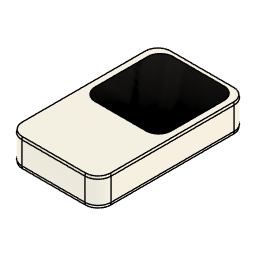
powerbank (Autodesk Fusion 360 design; units mm, degrees)
part number: 2025-04-07-12-48-19-748
Autodesk Fusion 360 part; units mm, degrees
note: some values were not read from the file. Chosen so that the rebuilt part matches the saved one: which bodies a step acts on.
sketch "Szkic1" plane through (0, 0, 0) normal (0, 0, 1) x (1, 0, 0)
  line L0 (-25, 58.75) -> (25, 58.75)
  line L1 (35, 48.75) -> (35, -48.75)
  line L2 (25, -58.75) -> (-25, -58.75)
  line L3 (-35, -48.75) -> (-35, 48.75)
  line L4 (-35, 58.75) -> (35, -58.75) construction
  line L5 (35, 58.75) -> (-35, -58.75) construction
  arc A0 (35, 48.75) -> (25, 58.75) centre (25, 48.75) ccw
  arc A1 (-25, 58.75) -> (-35, 48.75) centre (-25, 48.75) ccw
  arc A2 (-35, -48.75) -> (-25, -58.75) centre (-25, -48.75) ccw
  arc A3 (25, -58.75) -> (35, -48.75) centre (25, -48.75) ccw
  dimension "d1" = 70
  dimension "d2" = 117.5
  dimension "d3" = 10
  constraint horizontal L0
  constraint perpendicular L0 L1
  constraint parallel L0 L2
  constraint parallel L1 L3
  constraint coincident L4 origin
  constraint coincident L5 origin
  constraint coincident L5.start L1
  constraint coincident L5.start L0
  constraint tangent L1 A0
  constraint tangent L0 A0
  constraint coincident L4.start L0
  constraint coincident L4.start L3
  constraint tangent L0 A1
  constraint tangent L3 A1
  constraint equal A0 A1
  constraint coincident L5.end L3
  constraint coincident L5.end L2
  constraint tangent L3 A2
  constraint tangent L2 A2
  constraint equal A0 A2
  constraint coincident L4.end L2
  constraint coincident L4.end L1
  constraint tangent L2 A3
  constraint tangent L1 A3
  constraint equal A0 A3
  measures "d1" distance of L4.end L5.end
  measures "d2" distance of L5.start L4.end
  measures "d3" radius of A0
extrude "Wyciągnięcie proste4" add sketch "Szkic1" along normal blind 2 draft 10 makes body 1
extrude "Wyciągnięcie proste5" add 1 faces at (11.7842, -16.25, 2) along direction (0, 0, 1) blind 18 on bodies 1 bodies 1
extrude "Wyciągnięcie proste6" add 1 faces at (11.7842, -16.25, 20) along direction (0, 0, 1) blind 2 draft -10 on bodies 1 bodies 1
sketch "Szkic3" plane through (0, 0, 22) normal (0, 0, 1) x (-1, 0, 0)
  line L0 (35, -48.75) -> (35, 48.75)
  arc A0 (35, 48.75) -> (25, 58.75) centre (25, 48.75) ccw
  line L1 (25, 58.75) -> (-25, 58.75)
  arc A1 (-25, 58.75) -> (-35, 48.75) centre (-25, 48.75) ccw
  line L2 (-35, 48.75) -> (-35, -48.75)
  arc A2 (-35, -48.75) -> (-25, -58.75) centre (-25, -48.75) ccw
  line L3 (-25, -58.75) -> (25, -58.75)
  arc A3 (25, -58.75) -> (35, -48.75) centre (25, -48.75) ccw
  line L4 (-20.1713, -55.8211) -> (20.1713, -55.8211)
  line L5 (30.1713, -45.8211) -> (30.1713, -4.1789)
  line L6 (20.1713, 5.8211) -> (-20.1713, 5.8211)
  line L7 (-30.1713, -4.1789) -> (-30.1713, -45.8211)
  line L8 (-30.1713, -55.8211) -> (30.1713, 5.8211) construction
  line L9 (30.1713, -55.8211) -> (-30.1713, 5.8211) construction
  arc A4 (20.1713, -55.8211) -> (30.1713, -45.8211) centre (20.1713, -45.8211) ccw
  arc A5 (-30.1713, -45.8211) -> (-20.1713, -55.8211) centre (-20.1713, -45.8211) ccw
  arc A6 (-20.1713, 5.8211) -> (-30.1713, -4.1789) centre (-20.1713, -4.1789) ccw
  arc A7 (30.1713, -4.1789) -> (20.1713, 5.8211) centre (20.1713, -4.1789) ccw
  point P0 (0, -25)
  dimension "d23" = 10
  constraint horizontal L4
  constraint perpendicular L4 L5
  constraint parallel L4 L6
  constraint parallel L5 L7
  constraint coincident L8 P0
  constraint coincident L9 P0
  constraint coincident L9.start L5
  constraint coincident L9.start L4
  constraint tangent L5 A4
  constraint tangent L4 A4
  constraint coincident L8.start L4
  constraint coincident L8.start L7
  constraint tangent L4 A5
  constraint tangent L7 A5
  constraint equal A4 A5
  constraint coincident L9.end L7
  constraint coincident L9.end L6
  constraint tangent L7 A6
  constraint tangent L6 A6
  constraint equal A4 A6
  constraint coincident L8.end L5
  constraint coincident L8.end L6
  constraint tangent L5 A7
  constraint tangent L6 A7
  constraint equal A4 A7
  measures "d23" radius of A4
split "Podział1" by curves path "Szkic3" along L7 A5 L4 A4 L5 A7 L6 A6 bodies 1 makes body 2 at (-6.7238, -41.107, 22)
sketch "Szkic4" plane through (0, 59.1027, 0) normal (0, 1, 0) x (-1, 0, 0)
  line L0 (-25, 2) -> (25, 2)
  line L1 (25, 2) -> (25, 20)
  line L2 (25, 20) -> (-25, 20)
  line L3 (-25, 20) -> (-25, 2)
  line L4 (24, 6) -> (6, 6)
  line L5 (6, 6) -> (6, 14)
  line L6 (6, 14) -> (24, 14)
  line L7 (24, 14) -> (24, 6)
  line L8 (24, 6) -> (6, 14) construction
  line L9 (6, 6) -> (24, 14) construction
  line L10 (-20, 11) -> (-10, 11)
  line L11 (-10, 11) -> (-10, 9)
  line L12 (-10, 9) -> (-20, 9)
  line L13 (-20, 9) -> (-20, 11)
  line L14 (-20, 11) -> (-10, 9) construction
  line L15 (-10, 11) -> (-20, 9) construction
  line L16 (-7, 11) -> (3, 11)
  line L17 (3, 11) -> (3, 9)
  line L18 (3, 9) -> (-7, 9)
  line L19 (-7, 9) -> (-7, 11)
  line L20 (-7, 11) -> (3, 9) construction
  line L21 (3, 11) -> (-7, 9) construction
  point P0 (15, 10)
  point P1 (-15, 10)
  point P2 (-2, 10)
  constraint horizontal L4
  constraint perpendicular L4 L5
  constraint parallel L4 L6
  constraint parallel L5 L7
  constraint coincident L8 P0
  constraint coincident L9 P0
  constraint horizontal L10
  constraint perpendicular L10 L11
  constraint parallel L10 L12
  constraint parallel L11 L13
  constraint coincident L14 P1
  constraint coincident L15 P1
  constraint horizontal L16
  constraint perpendicular L16 L17
  constraint parallel L16 L18
  constraint parallel L17 L19
  constraint coincident L20 P2
  constraint coincident L21 P2
extrude "Wyciągnięcie proste7" cut sketch "Szkic4" against normal blind 4 contours L4 L5 L6 L7 | L10 L11 L12 L13 | L16 L17 L18 L19 bodies 1 2
sketch "Szkic5" plane through (-35.3527, 0, 0) normal (-1, 0, 0) x (0, -1, 0)
  line L0 (-48.75, 2) -> (48.75, 2)
  line L1 (48.75, 2) -> (48.75, 20)
  line L2 (48.75, 20) -> (-48.75, 20)
  line L3 (-48.75, 20) -> (-48.75, 2)
  line L4 (-45, 15) -> (-40, 15)
  line L5 (-40, 15) -> (-40, 5)
  line L6 (-40, 5) -> (-45, 5)
  line L7 (-45, 5) -> (-45, 15)
  line L8 (-30, 13) -> (-19, 13)
  line L9 (-19, 13) -> (-19, 8)
  line L10 (-19, 8) -> (-30, 8)
  line L11 (-30, 8) -> (-30, 13)
  line L12 (0, 15) -> (27, 15)
  line L13 (27, 15) -> (27, 6)
  line L14 (27, 6) -> (0, 6)
  line L15 (0, 6) -> (0, 15)
  constraint horizontal L4
  constraint vertical L5
  constraint horizontal L6
  constraint vertical L7
  constraint horizontal L8
  constraint vertical L9
  constraint horizontal L10
  constraint vertical L11
  constraint horizontal L12
  constraint vertical L13
  constraint horizontal L14
  constraint vertical L15
extrude "Wyciągnięcie proste8" cut sketch "Szkic5" against normal blind 5 contours L4 L5 L6 L7 | L8 L9 L10 L11 | L12 L13 L14 L15 bodies 2
sketch "Szkic6" plane through (0, 19, 0) normal (0, 1, 0) x (-1, 0, 0)
  line L0 (35.3527, 8) -> (35.3527, 13)
  line L1 (35.3527, 13) -> (30.3527, 13)
  line L2 (30.3527, 13) -> (30.3527, 8)
  line L3 (30.3527, 8) -> (35.3527, 8)
  line L4 (30.3527, 12.4932) -> (32.6473, 12.4932)
  line L5 (32.6473, 12.4932) -> (32.6473, 7.5068)
  line L6 (32.6473, 7.5068) -> (30.3527, 7.5068)
  line L7 (30.3527, 7.5068) -> (30.3527, 12.4932)
  line L8 (30.3527, 12.4932) -> (32.6473, 7.5068) construction
  line L9 (32.6473, 12.4932) -> (30.3527, 7.5068) construction
  point P0 (31.5, 10)
  constraint horizontal L4
  constraint perpendicular L4 L5
  constraint parallel L4 L6
  constraint parallel L5 L7
  constraint coincident L8 P0
  constraint coincident L9 P0
  constraint coincident L2 L4.start
extrude "Wyciągnięcie proste9" cut sketch "Szkic6" against normal blind 30 contours L2 L3 L4 L5 L7 bodies 2
